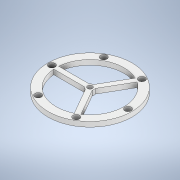
# Autodesk Inventor part: reaction wheel
Saved by Autodesk Inventor 2021 (Build 250183000, 183)
## iProperties
Created: 2021-07-30
Part Number: reaction wheel
Material: PC/ABS Plastic
Document SubType Name: Modeling
Designer: samlo
Density: 0.357273 g/cm^3
Appearance: Smooth - White
Mass: 7.13487 g
Surface Area: 124.858 cm^2
Volume: 19.9704 cm^3
Author: samlo
Autodesk Inventor part; units mm, degrees
ref_plane "YZ Plane" through (0, 0, 0) normal (1, 0, 0) x (0, 1, 0)
ref_plane "XZ Plane" through (0, 0, 0) normal (0, 1, 0) x (-1, 0, 0)
ref_plane "XY Plane" through (0, 0, 0) normal (0, 0, 1) x (1, 0, 0)
sketch "Sketch1" plane through (0, 0, 0) normal (0, 1, 0) x (-1, 0, 0)
  circle A0 centre (0, 0) radius 51.45
  circle A1 centre (0, 0) radius 3
  line L0 (4, -3) -> (43.45, -3)
  line L1 (0.5981, 4.9641) -> (-19.1269, 39.1288)
  line L2 (-4.5981, -1.9641) -> (-24.3231, -36.1288)
  line L3 (4, 3) -> (43.45, 3)
  line L4 (-4.5981, 1.9641) -> (-24.3231, 36.1288)
  line L5 (0.5981, -4.9641) -> (-19.1269, -39.1288)
  arc A2 (4, 3) -> (0.5981, 4.9641) centre (0, 0) ccw
  arc A3 (-4.5981, 1.9641) -> (-4.5981, -1.9641) centre (0, 0) ccw
  arc A4 (0.5981, -4.9641) -> (4, -3) centre (0, 0) ccw
  arc A5 (-23.2687, 34.3026) -> (-23.2687, -34.3026) centre (0, 0) ccw
  arc A6 (-18.0726, -37.3026) -> (41.3413, -3) centre (0, 0) ccw
  arc A7 (41.3413, 3) -> (-18.0726, 37.3026) centre (0, 0) ccw
  circle A8 centre (-23.127, -40.341) radius 4
  circle A9 centre (23.3728, -40.199) radius 4
  circle A10 centre (46.4998, 0.1419) radius 4
  circle A11 centre (23.127, 40.341) radius 4
  circle A12 centre (-23.3728, 40.199) radius 4
  circle A13 centre (-46.4998, -0.1419) radius 4
  dimension "d0" = 102.9
  dimension "d2" = 6
  dimension "d7" = 360
  dimension "d9" = 6
  dimension "d12" = 360
  dimension "d16" = 8
  dimension "d17" = 46.5
  dimension "d20" = 360
  constraints: 14 centre point, 12 end point, 12 point on circle, 6 point on line, 4 coincident, 1 parallel, 33 other
  measures "d0" diameter of A0
  measures "d2" diameter of A1
  measures "d9" distance between parallel lines of L0 L3
  measures "d16" diameter of A8
  measures "d17" distance of point (0, 0) A8.centre
extrude "Extrusion2" add sketch "Sketch1" along normal blind 6
body "Solid2"
